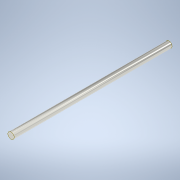
# Autodesk Inventor part: Varilla 200
Saved by Autodesk Inventor 2022 (Build 260153000, 153)
## iProperties
Created: 2021-11-08
Part Number: Varilla 200
Material: Steel
Document SubType Name: Modeling
Designer: Samuel Gómez
Mass: 78.9168 g
Surface Area: 51.2708 cm^2
Volume: 10.0531 cm^3
Density: 7.85 g/cm^3
Appearance: Silver
Author: Samuel Gómez
Autodesk Inventor part; units mm, degrees
ref_plane "YZ Plane" through (0, 0, 0) normal (1, 0, 0) x (0, 1, 0)
ref_plane "XZ Plane" through (0, 0, 0) normal (0, 1, 0) x (-1, 0, 0)
ref_plane "XY Plane" through (0, 0, 0) normal (0, 0, 1) x (1, 0, 0)
sketch "Boceto1" plane through (0, 0, 0) normal (0, 0, 1) x (1, 0, 0)
  circle A0 centre (0, 0) radius 4
  dimension "d0" = 8
  constraints: 1 centre point, 1 coincident
  measures "d0" diameter of A0
extrude "Extrusión1" add sketch "Boceto1" along normal blind 200
